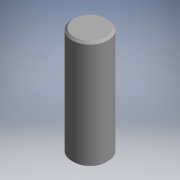
# Autodesk Inventor part: D-51
Saved by Autodesk Inventor 2017.3 (Build 213256000, 256)
## iProperties
Part Number: D-51
Material: Generic
Catalog Web Link: www.cadenas.de
Description: Pin-Original Line - Standard Air Cylinders
Vendor: BIMBA
Document SubType Name: Modeling
Designer: partserver
Manufacturer: BIMBA
Mass: 0.60147 g
Surface Area: 4.36028 cm^2
Volume: 0.60147 cm^3
Density: 1 g/cm^3
Appearance: PSOLRGB-192-192-192
Category: PARTsolutions
Company: BIMBA
Title: D-51
Author: Cadenas PARTsolutions
Comments: Original Line - Standard Air Cylinders
PSOL_IDENT_0: {$CADENAS_DATA\23d-libs\bimba\bimba_brand\bimba_imperial\bimba_full_line\original_line_cylinders\sta
PSOL_IDENT_1: ndard_air_cylinders\pin.prj},145 {VTYP=3D},{NB=D-51},{LINA=D-51},{NN=Pin},{DATE=19.01.2022 10:19:37}
PSOL_IDENT_2: ,{GEOMDATE=15.02.2011 00:00:00},{VERSION=},{LINEID=10},{WBVAR=},{WBNUMERIC=}  {NB=D-51},{LINA=D-51},
PSOL_IDENT_3: {KT=DUMMY},{PN=D-51},{DIA=0.25000},{L=0.7500}
NB: D-51
NN: Pin
NT: Original Line - Standard Air Cylinders
NBSYN: $PN.
LINA: D-51
CATALOG: Bimba Products
PN: D-51
DIA: 0.25
L: 0.75
SUPPLIER: BIMBA
ARTICLENO: D-51
BOMINFO: D-51
CREATOR: CADENAS GmbH
Autodesk Inventor part; units mm, degrees
sketch "Sketch_1" plane through (0, 0, 0) normal (1, 0, 0) x (0, 1, 0)
  line L0 (0, -9.525) -> (0, 9.525)
  line L1 (0, 9.525) -> (2.9236, 9.525)
  line L2 (2.9236, 9.525) -> (3.175, 9.2736)
  line L3 (3.175, 9.2736) -> (3.175, -9.1694)
  line L4 (3.175, -9.1694) -> (2.8194, -9.525)
  line L5 (2.8194, -9.525) -> (0, -9.525)
  line L6 (0, -9.525) -> (0, 9.525)
  constraints: 14 end point
revolve "Revolution1" add sketch "Sketch_1" angle 360 about axis through (0, 0, -9.525) along (0, 0, -1)
ref_plane "dia1_XY" through (-3.175, 0, 0) normal (0, 0, 1) x (1, 0, 0)
ref_plane "dia1_YZ" through (-3.175, 0, 0) normal (1, 0, 0) x (0, 1, 0)
ref_plane "dia1_ZX" through (-3.175, 0, 0) normal (0, 1, 0) x (0, 0, 1)
ref_plane "dia2_XY" through (3.175, 0, 0) normal (0, 0, 1) x (1, 0, 0)
ref_plane "dia2_YZ" through (3.175, 0, 0) normal (1, 0, 0) x (0, 1, 0)
ref_plane "dia2_ZX" through (3.175, 0, 0) normal (0, 1, 0) x (0, 0, 1)
ref_plane "pin_XY" through (0, 0, 0) normal (0, 0, 1) x (1, 0, 0)
ref_plane "pin_YZ" through (0, 0, 0) normal (1, 0, 0) x (0, 1, 0)
ref_plane "pin_ZX" through (0, 0, 0) normal (0, 1, 0) x (0, 0, 1)
ref_plane "pin1_XY" through (0, 0, 9.525) normal (1, 0, 0) x (0, 0, -1)
ref_plane "pin1_YZ" through (0, 0, 9.525) normal (0, 0, -1) x (0, 1, 0)
ref_plane "pin1_ZX" through (0, 0, 9.525) normal (0, 1, 0) x (1, 0, 0)
ref_plane "pin2_XY" through (0, 0, -9.525) normal (1, 0, 0) x (0, 0, -1)
ref_plane "pin2_YZ" through (0, 0, -9.525) normal (0, 0, -1) x (0, 1, 0)
ref_plane "pin2_ZX" through (0, 0, -9.525) normal (0, 1, 0) x (1, 0, 0)
body "Solid1"
